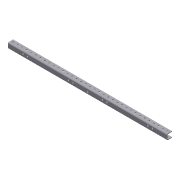
# Autodesk Inventor part: C Channel
Saved by Autodesk Inventor 2011 (Build 150239000, 239)
## iProperties
Created: 2012-01-09
Part Number: C Channel
Material: Aluminum-5052
Document SubType Name: Sheet Metal
Designer: Nemo
Density: 2.67941 g/cm^3
Flat Pattern Width: 7.78634 cm
Flat Pattern Length: 88.9 cm
Flat Pattern Area: 692.205 cm^2
Sheet Metal Rule: 0.125 Aluminum-5052
Sheet Metal Width: 3.065 in
Sheet Metal Length: 35.000 in
Sheet Metal Area: 107.292 in^2
Author: Nemo
Autodesk Inventor part; units mm, degrees
ref_plane "YZ Plane" through (0, 0, 0) normal (1, 0, 0) x (0, 1, 0)
ref_plane "XZ Plane" through (0, 0, 0) normal (0, 1, 0) x (-1, 0, 0)
ref_plane "XY Plane" through (0, 0, 0) normal (0, 0, 1) x (1, 0, 0)
sketch "Sketch3" plane through (0, 0, 0) normal (0, 0, 1) x (1, 0, 0)
  line L0 (-444.5, 9.525) -> (444.5, 9.525)
  line L1 (444.5, 9.525) -> (444.5, -9.525)
  line L2 (444.5, -9.525) -> (-444.5, -9.525)
  line L3 (-444.5, -9.525) -> (-444.5, 9.525)
  point P0 (0, 0)
  point P1 (-444.5, 0)
  point P2 (0, 9.525)
  dimension "d3" = 889
  dimension "d4" = 19.05
  measures "d3" distance of L0.start L0.end
  measures "d4" distance of L2.end L0.start
extrude "Plate2" add sketch "Sketch3" along normal blind 3.175
sketch "Sketch4" plane through (444.5, 12.7, -3.175) normal (0, 1, 0) x (-1, 0, 0)
  line L0 (889, 0) -> (0, 0)
  line L1 (0, 0) -> (0, -22.225)
  line L2 (0, -22.225) -> (889, -22.225)
  line L3 (889, -22.225) -> (889, 0)
  constraints: 4 end point, 4 other
edge flange "Flange1" height 28.575 angle 90 thickness 3.175 bend radius 3.175 thickness toward (0, 1, 0) relief straight relief width 3.175 relief depth 1.5875 corner gap 3.175 corner form 0 edges at (0, 9.525, 0) (0, -9.525, 0) wall of the first edge with corners at (-444.5, 12.7, -3.175) (444.5, 12.7, -3.175) (444.5, 12.7, -25.4) (-444.5, 12.7, -25.4)
bend "Bend1"
corner "Corner1"
sketch "Sketch1" plane through (0, 0, 0) normal (0, 0, 1) x (1, 0, 0)
  line L0 (0, 0) -> (0, 77.8634) projected
  line L1 (889, 0) -> (0, 0) projected
  line L2 (889, 77.8634) -> (889, 0) projected
  line L3 (0, 77.8634) -> (889, 77.8634) projected
unfold all bends "Unfold1" k factor 0.44 fixed face at (-148.1667, 3.175, 3.175)
sketch "Sketch6" plane through (0, 0, 3.175) normal (0, 0, 1) x (1, 0, 0)
  line L0 (444.5, 9.525) -> (444.5, -9.525) projected
  line L1 (-444.5, -9.525) -> (-444.5, 9.525) projected
  line L2 (-444.5, 16.7067) -> (444.5, 16.7067) projected
  line L3 (444.5, 38.9317) -> (444.5, 16.7067) projected
  line L4 (-444.5, 38.9317) -> (444.5, 38.9317) projected
  line L5 (-444.5, 16.7067) -> (-444.5, 38.9317) projected
  line L6 (-444.5, 16.7067) -> (444.5, 16.7067) projected
  line L7 (-444.5, 9.525) -> (-444.5, 16.7067) projected
  line L8 (-444.5, 9.525) -> (444.5, 9.525) projected
  line L9 (444.5, 16.7067) -> (444.5, 9.525) projected
  line L10 (444.5, -16.7067) -> (-444.5, -16.7067) projected
  line L11 (-444.5, -38.9317) -> (-444.5, -16.7067) projected
  line L12 (444.5, -38.9317) -> (-444.5, -38.9317) projected
  line L13 (444.5, -16.7067) -> (444.5, -38.9317) projected
  line L14 (444.5, -16.7067) -> (-444.5, -16.7067) projected
  line L15 (444.5, -9.525) -> (444.5, -16.7067) projected
  line L16 (444.5, -9.525) -> (-444.5, -9.525) projected
  line L17 (-444.5, -16.7067) -> (-444.5, -9.525) projected
  line L18 (-444.5, 0) -> (444.5, 0) construction
  point P0 (0, 0)
  point P1 (-431.8, 26.2317)
  point P2 (-431.8, -26.2317)
  dimension "d19" = 12.7
  dimension "d20" = 12.7
  dimension "d21" = 12.7
  dimension "d22" = 12.7
  constraints: 2 end point, 2 midpoint
  measures "d19" distance from line of point (-431.8, 26.232) L5
  measures "d20" distance from line of L11 point (-431.8, -26.232)
  measures "d21" distance from line of L12 point (-431.8, -26.232)
  measures "d22" distance from line of L4 point (-431.8, 26.232)
hole "Hole1" at (-431.8, 26.2317, 3.175) at (-431.8, -26.2317, 3.175) direction (0, 0, -1) diameter 6.5278 depth 3.175 tip angle 118
pattern_linear "Rectangular Pattern1" count 35 spacing 25.4 along (1, 0, 0) of "Hole1"
sketch "Sketch7" plane through (0, 0, 3.175) normal (0, 0, 1) x (1, 0, 0)
  line L0 (-444.5, -9.525) -> (-444.5, 9.525) projected
  line L1 (444.5, -9.525) -> (-444.5, -9.525) projected
  line L2 (-444.5, 38.9317) -> (444.5, 38.9317) projected
  line L3 (-444.5, 16.7067) -> (-444.5, 38.9317) projected
  line L4 (0, 38.9317) -> (0, -9.525) construction
  point P0 (0, 0)
  point P1 (-361.95, -1.9115)
  point P2 (-82.55, -1.9115)
  point P3 (-336.55, -1.9115)
  point P4 (-107.95, -1.9115)
  point P5 (0, 1.8985)
  point P6 (361.95, -1.9115)
  point P7 (82.55, -1.9115)
  point P8 (336.55, -1.9115)
  point P9 (107.95, -1.9115)
  dimension "d33" = 82.55
  dimension "d34" = 107.95
  dimension "d35" = 336.55
  dimension "d36" = 361.95
  dimension "d37" = 37.0332
  dimension "d38" = 40.8432
  constraints: 4 symmetric about line, 3 horizontal alignment, 2 end point, 2 midpoint, 1 vertical alignment
  measures "d33" distance from line of point (-361.95, -1.912) L0
  measures "d34" distance from line of L0 point (-336.55, -1.912)
  measures "d35" distance from line of L0 point (-107.95, -1.912)
  measures "d36" distance from line of L0 point (-82.55, -1.912)
  measures "d37" distance from line of L2 point (0, 1.898)
  measures "d38" distance from line of point (-361.95, -1.912) L2
hole "Hole2" at (-361.95, -1.9115, 3.175) at (-82.55, -1.9115, 3.175) at (-336.55, -1.9115, 3.175) at (-107.95, -1.9115, 3.175) at (0, 1.8985, 3.175) at (361.95, -1.9115, 3.175) at (336.55, -1.9115, 3.175) at (107.95, -1.9115, 3.175) at (82.55, -1.9115, 3.175) direction (0, 0, -1) diameter 9.652 depth 3.175 tip angle 118
refold all bends "Refold1"
ref_plane "Work Plane1" through (0, -9.525, 0) normal (-1, 0, 0) x (0, 0, 1)
equation "\"d28\" = Thickness"
equation "\"d44\" = Thickness"
equation "\"d6\" = BendReliefWidth"
equation "\"d7\" = BendReliefDepth"
equation "\"d8\" = MinimumRemnant"
equation "\"d9\" = BendRadius"
equation "\"d12\" = BendRadius"
equation "\"d13\" = CornerReliefSize"
equation "\"d14\" = GapSize"
equation "\"d15\" = JacobiRadiusSize"
equation "\"BendRadius\" = Thickness"
equation "\"BendReliefWidth\" = Thickness"
equation "\"BendReliefDepth\" = 0.5 * Thickness"
equation "\"CornerReliefSize\" = 4 * Thickness"
equation "\"MinimumRemnant\" = 2 * Thickness"
equation "\"TransitionRadius\" = BendRadius"
equation "\"JacobiRadiusSize\" = BendRadius"
equation "\"GapSize\" = Thickness"
equation "\"d2\" = BendRadius"
equation "\"d5\" = BendRadius"
equation "\"Thickness\" = 3.175"
body "Solid2"
